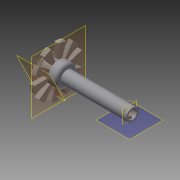
# Autodesk Inventor part: axiel
Saved by Autodesk Inventor 2015 (Build 190159000, 159)
## iProperties
Created: 2015-12-15
Part Number: axiel
Material: Generic
Document SubType Name: Modeling
Designer: Ross
Density: 1 g/cm^3
Appearance: Default
Author: Ross
Autodesk Inventor part; units mm, degrees
ref_plane "XZ Plane" through (0, 0, 0) normal (0, 1, 0) x (-1, 0, 0)
ref_plane "XY Plane" through (0, 0, 0) normal (0, 0, 1) x (1, 0, 0)
sketch "Sketch1" plane through (0, 0, 0) normal (1, 0, 0) x (0, 1, 0)
  arc A0 (16, 0) -> (15.2169, 4.9443) centre (0, 0) ccw
  line L0 (0, 0) -> (15.2169, 4.9443) construction
  line L1 (0, 0) -> (16, 0) construction
  line L2 (0, 0) -> (15.2169, 4.9443) construction
  line L3 (15.2169, 4.9443) -> (0, 0)
  line L4 (16, 0) -> (0, 0)
  arc A1 (16, 0) -> (15.2169, 4.9443) centre (0, 0) ccw
  dimension "d0" = 16
  dimension "d1" = 18
  constraints: 10 end point, 4 point on circle, 3 coincident, 2 centre point, 1 collinear, 1 horizontal
  measures "d0" radius of A0
  measures "d1" angle of L1 L0
extrude "Extrusion1" add sketch "Sketch1" along normal blind 3
pattern_circular "Circular Pattern1" count 10 over 360 about axis through (-10, 0, 0) along (1, 0, 0) of "Extrusion1"
ref_plane "Work Plane1" through (3, 0, 0) normal (1, 0, 0) x (0, 1, 0)
sketch "Sketch2" plane through (0, 0, 0) normal (1, 0, 0) x (0, 1, 0)
  circle A0 centre (0, 0) radius 7
  dimension "d9" = 14
  constraints: 1 centre point, 1 coincident
  measures "d9" diameter of A0
extrude "Extrusion2" add sketch "Sketch2" against normal blind 4.5
sketch "Sketch3" plane through (3, 0, 0) normal (1, 0, 0) x (0, 1, 0)
  circle A0 centre (0, 0) radius 7
  point P0 (0, -7)
  constraints: 1 coincident, 1 vertical alignment, 2 other
extrude "Extrusion3" add sketch "Sketch3" against normal blind 3
sketch "Sketch4" plane through (3, 0, 0) normal (1, 0, 0) x (0, 0, -1)
  circle A0 centre (0, 0) radius 7
  constraints: 1 centre point, 1 coincident
extrude "Extrusion4" add sketch "Sketch4" along normal blind 4.5
sketch "Sketch5" plane through (7.5, 0, 0) normal (1, 0, 0) x (0, 0, -1)
  circle A0 centre (0, 0) radius 4.1
  dimension "d16" = 8.2
  constraints: 1 centre point, 1 coincident
  measures "d16" diameter of A0
extrude "Extrusion5" add sketch "Sketch5" along normal blind 40
sketch "Sketch6" plane through (-4.5, 0, 0) normal (-1, 0, 0) x (0, 0, 1)
  circle A0 centre (0, 0) radius 0.925
  dimension "d19" = 1.85
  constraints: 1 centre point, 1 coincident
  measures "d19" diameter of A0
extrude "Extrusion6" cut sketch "Sketch6" against normal blind 9
sketch "Sketch7" plane through (7.5, 0, 0) normal (1, 0, 0) x (0, 0, -1)
  circle A0 centre (0, 0) radius 7
  constraints: 1 centre point, 1 coincident
extrude "Extrusion7" add sketch "Sketch7" along normal blind 1
fillet "Fillet1" radius 2 1 edges at (8.5, 0, 7)
sketch "Sketch8" plane through (47.5, 0, 0) normal (1, 0, 0) x (0, 0, -1)
  circle A0 centre (0, 0) radius 2.9
  dimension "d25" = 5.8
  constraints: 1 centre point, 1 coincident
  measures "d25" diameter of A0
extrude "Extrusion8" cut sketch "Sketch8" against normal blind 40
sketch "Sketch9" plane through (47.5, 0, 0) normal (1, 0, 0) x (0, 0, -1)
  circle A0 centre (0, 0) radius 0.925 projected
  circle A1 centre (0, 0) radius 2.9
  circle A2 centre (0, 0) radius 4.1
  constraints: 2 centre point, 2 coincident
extrude "Extrusion9" add sketch "Sketch9" along normal blind 4 contours A2
ref_plane "Work Plane2" through (49.5, 0, 0) normal (1, 0, 0) x (0, 0, -1)
sketch "Sketch10" plane through (49.5, 0, 0) normal (1, 0, 0) x (0, 0, -1)
  line L0 (0, 0) -> (4.1, 0)
  circle A0 centre (0, 0) radius 4.1 projected
  constraints: 2 end point, 1 horizontal, 1 horizontal alignment, 1 other
ref_plane "Work Plane3" through (49.5, 0, -4.1) normal (0, 0, -1) x (-1, 0, 0)
sketch "Sketch11" plane through (49.5, 0, -4.1) normal (0, 0, -1) x (-1, 0, 0)
  circle A0 centre (0, 0) radius 1.25
  point P0 (49.5, 0)
  dimension "d31" = 2.5
  constraints: 1 centre point
  measures "d31" diameter of A0
sweep "Sweep1" cut profiles "Sketch11" path "Sketch10" path curves L0
ref_plane "Work Plane4" through (-2.5, 0, 0) normal (-1, 0, 0) x (0, 0, 1)
sketch "Sketch12" plane through (-2.5, 0, 0) normal (-1, 0, 0) x (0, 0, 1)
  circle A0 centre (0, 0) radius 7 projected
  line L0 (-3.1108, -6.2708) -> (-2.222, -4.4791)
  circle A1 centre (0, 0) radius 5 projected
  line L1 (0, 0) -> (-2.222, -4.4791)
  dimension "d35" = 2
  constraints: 4 end point, 4 other
  measures "d35" distance of L0.start L0.end
ref_plane "Work Plane5" through (-2.5, -6.2708, -3.1108) normal (0, -0.8958262, -0.4444046) x (1, 0, 0)
sketch "Sketch13" plane through (-2.5, -6.2708, -3.1108) normal (0, -0.8958262, -0.4444046) x (1, 0, 0)
  circle A0 centre (0, 0) radius 1.5
  point P0 (2.5, 0)
  dimension "d36" = 3
  constraints: 1 centre point
  measures "d36" diameter of A0
sweep "Sweep2" cut profiles "Sketch13" path "Sketch12" path curves L0
sketch "Sketch14" plane through (-2.5, 0, 0) normal (-1, 0, 0) x (0, 0, 1)
  line L0 (0, 0) -> (-2.222, -4.4791)
  line L1 (-0.8783, -5.1457) -> (-3.5658, -3.8125) projected
  constraints: 2 end point, 1 midpoint
sketch "Sketch15" plane through (-2.5, -4.4791, -2.222) normal (0, -0.8958262, -0.4444046) x (1, 0, 0)
  circle A0 centre (0, 0) radius 0.8
  point P0 (2.5, 0)
  dimension "d39" = 1.6
  constraints: 1 centre point
  measures "d39" diameter of A0
extrude "Extrusion10" cut sketch "Sketch15" against normal blind 5
pattern_circular "Circular Pattern2" count 3 over 360 about axis through (-10, 0, 0) along (1, 0, 0) of "Sweep2", "Extrusion10"
body "Solid1"
